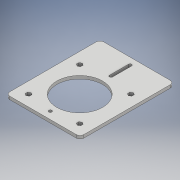
# Autodesk Inventor part: Адаптер для считывателя Bolid Proxy-2MA часть 2
Saved by Autodesk Inventor 2018 (Build 220112000, 112)
## iProperties
Created: 2019-06-30
Part Number: Адаптер для считывателя Bolid Proxy-2MA часть 2
Material: Типовые
Document SubType Name: Modeling
Designer: KV33_HP1
Density: 1 g/cm^3
Appearance: По умолчанию
Author: KV33_HP1
Autodesk Inventor part; units mm, degrees
ref_plane "YZ Plane" through (0, 0, 0) normal (1, 0, 0) x (0, 1, 0)
ref_plane "XZ Plane" through (0, 0, 0) normal (0, 1, 0) x (-1, 0, 0)
ref_plane "XY Plane" through (0, 0, 0) normal (0, 0, 1) x (1, 0, 0)
sketch "Эскиз1" plane through (0, 0, 0) normal (0, 0, 1) x (1, 0, 0)
  line L0 (5, 0) -> (92, 0)
  line L1 (97, 5) -> (97, 118)
  line L2 (92, 123) -> (5, 123)
  line L3 (0, 118) -> (0, 5)
  circle A0 centre (48.5, 48) radius 30
  arc A1 (5, 123) -> (0, 118) centre (5, 118) ccw
  arc A2 (97, 118) -> (92, 123) centre (92, 118) ccw
  arc A3 (92, 0) -> (97, 5) centre (92, 5) ccw
  arc A4 (0, 5) -> (5, 0) centre (5, 5) ccw
  arc A5 (46.5, 89) -> (50.5, 89) centre (48.5, 89) ccw
  arc A6 (50.5, 114) -> (46.5, 114) centre (48.5, 114) ccw
  line L4 (46.5, 89) -> (46.5, 114)
  line L5 (50.5, 114) -> (50.5, 89)
  circle A7 centre (48.5, 9.5) radius 2
  line L6 (12.1435, 79.8578) -> (12.1496, 83.1527)
  line L7 (12.1496, 83.1527) -> (15.0061, 84.7949)
  line L8 (15.0061, 84.7949) -> (17.8565, 83.1422)
  line L9 (17.8565, 83.1422) -> (17.8504, 79.8473)
  line L10 (17.8504, 79.8473) -> (14.9939, 78.2051)
  line L11 (14.9939, 78.2051) -> (12.1435, 79.8578)
  line L12 (12.1435, 12.8578) -> (12.1496, 16.1527)
  line L13 (12.1496, 16.1527) -> (15.0061, 17.7949)
  line L14 (15.0061, 17.7949) -> (17.8565, 16.1422)
  line L15 (17.8565, 16.1422) -> (17.8504, 12.8473)
  line L16 (17.8504, 12.8473) -> (14.9939, 11.2051)
  line L17 (14.9939, 11.2051) -> (12.1435, 12.8578)
  line L18 (79.1435, 12.8578) -> (79.1496, 16.1527)
  line L19 (79.1496, 16.1527) -> (82.0061, 17.7949)
  line L20 (82.0061, 17.7949) -> (84.8565, 16.1422)
  line L21 (84.8565, 16.1422) -> (84.8504, 12.8473)
  line L22 (84.8504, 12.8473) -> (81.9939, 11.2051)
  line L23 (81.9939, 11.2051) -> (79.1435, 12.8578)
  line L24 (79.1435, 79.8578) -> (79.1496, 83.1527)
  line L25 (79.1496, 83.1527) -> (82.0061, 84.7949)
  line L26 (82.0061, 84.7949) -> (84.8565, 83.1422)
  line L27 (84.8565, 83.1422) -> (84.8504, 79.8473)
  line L28 (84.8504, 79.8473) -> (81.9939, 78.2051)
  line L29 (81.9939, 78.2051) -> (79.1435, 79.8578)
  point P0 (0, 0)
  point P1 (97, 123)
  point P2 (0, 123)
  point P3 (15, 81.5)
  point P4 (15, 14.5)
  point P5 (15, 14.5)
  point P6 (82, 14.5)
  point P7 (82, 14.5)
  point P8 (82, 81.5)
  point P9 (82, 81.5)
  dimension "d10" = 5
  dimension "d21" = 4
  dimension "d22" = 4
  dimension "d23" = 4
  constraints: 60 end point, 12 point on circle, 10 tangent, 8 centre point, 6 point on line, 3 equal radius, 3 parallel, 1 horizontal, 1 perpendicular, 1 vertical, 52 other
  measures "d10" radius of A1
  measures "d21" diameter of A5
  measures "d22" diameter of A6
  measures "d23" diameter of A7
extrude "Выдавливание1" add sketch "Эскиз1" along normal blind 4
